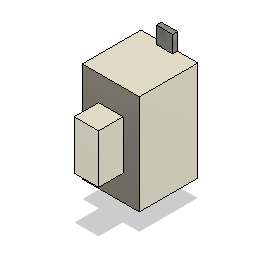
IR_MiniHolder_25mm_3mmLED_Resin (Autodesk Fusion 360 archive; units mm, degrees)
design "Switch"
Autodesk Fusion 360 part; units mm, degrees
sketch "Sketch1" plane through (0, 0, 0) normal (0, 0, 1) x (1, 0, 0)
  line L0 (1.75, 3.06) -> (-1.75, 3.06)
  line L1 (-1.75, 3.06) -> (-1.75, -3.06)
  line L2 (-1.75, -3.06) -> (1.75, -3.06)
  line L3 (1.75, -3.06) -> (1.75, 3.06)
  line L4 (1.75, 3.06) -> (-1.75, -3.06) construction
  line L5 (-1.75, 3.06) -> (1.75, -3.06) construction
  line L6 (0.75, 1.5) -> (-0.75, 1.5)
  line L7 (-0.75, 1.5) -> (-0.75, -1.5)
  line L8 (-0.75, -1.5) -> (0.75, -1.5)
  line L9 (0.75, -1.5) -> (0.75, 1.5)
  line L10 (0.75, 1.5) -> (-0.75, -1.5) construction
  line L11 (-0.75, 1.5) -> (0.75, -1.5) construction
  dimension "d1" = 3.5
  dimension "d2" = 6.12
  dimension "d3" = 1.5
  dimension "d4" = 3
  constraint horizontal L0
  constraint perpendicular L0 L1
  constraint parallel L0 L2
  constraint parallel L1 L3
  constraint coincident L4 origin
  constraint coincident L5 origin
  constraint horizontal L6
  constraint perpendicular L6 L7
  constraint parallel L6 L8
  constraint parallel L7 L9
  constraint coincident L10 origin
  constraint coincident L11 origin
  measures "d1" distance of L1.end L2.end
  measures "d2" distance of L0.end L1.end
  measures "d3" distance of L7.end L8.end
  measures "d4" distance of L6.end L7.end
extrude "Extrude1" add sketch "Sketch1" along normal blind 1.5 contours L6 L7 L8 L9 makes body 1
extrude "Extrude2" add sketch "Sketch1" against normal blind 3.6 separate body contours L0 L1 L2 L3 | L6 L7 L8 L9 makes body 2
sketch "Sketch2" plane through (0, 0, -3.6) normal (0, 0, -1) x (-1, 0, 0)
  line L0 (-1.75, 3.06) -> (-1.75, -3.06)
  line L1 (-1.75, -3.06) -> (1.75, -3.06)
  line L2 (1.75, -3.06) -> (1.75, 3.06)
  line L3 (1.75, 3.06) -> (-1.75, 3.06)
  line L4 (-0.5, 4.1) -> (0.5, 4.1)
  line L5 (0.5, 4.1) -> (0.5, -4.1)
  line L6 (0.5, -4.1) -> (-0.5, -4.1)
  line L7 (-0.5, -4.1) -> (-0.5, 4.1)
  line L8 (-0.5, 4.1) -> (0.5, -4.1) construction
  line L9 (0.5, 4.1) -> (-0.5, -4.1) construction
  dimension "d9" = 1
  dimension "d10" = 8.2
  constraint horizontal L4
  constraint perpendicular L4 L5
  constraint parallel L4 L6
  constraint parallel L5 L7
  constraint coincident L8 origin
  constraint coincident L9 origin
  measures "d9" distance of L5.end L6.end
  measures "d10" distance of L4.end L5.end
extrude "Extrude3" add sketch "Sketch2" against normal blind 0.3 separate body contours L3 L4 L5 L7 | L1 L5 L6 L7 makes body 3 at (0.1667, 3.7533, -3.6) makes body 4 at (0.1667, -3.4067, -3.6)
